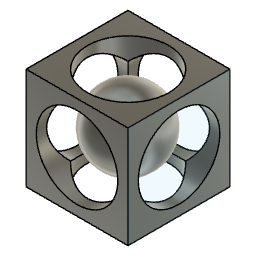
Sphere cube (Autodesk Fusion 360 design; units mm, degrees)
Autodesk Fusion 360 part; units mm, degrees
sketch "Sketch1" plane through (0, 0, 0) normal (0, 0, 1) x (1, 0, 0)
  line L0 (0, 25) -> (25, 25)
  line L1 (25, 25) -> (25, 0)
  line L2 (25, 0) -> (0, 0)
  line L3 (0, 0) -> (0, 25)
  constraint horizontal L0
  constraint perpendicular L0 L1
  constraint coincident L2.end L3.start
  constraint perpendicular L1 L2
  constraint perpendicular L0 L3
extrude "Extrude1" add sketch "Sketch1" along normal blind 25 makes body 1
sketch "Sketch2" plane through (0, 0, 0) normal (0, -1, 0) x (1, 0, 0)
  line L0 (0, 0) -> (25, 0)
  line L1 (25, 0) -> (25, 25)
  line L2 (25, 25) -> (0, 25)
  line L3 (0, 25) -> (0, 0)
  circle A0 centre (12.5, 12.5) radius 10
  dimension "d3" = 20
  measures "d3" diameter of A0
extrude "Extrude2" cut sketch "Sketch2" against normal blind 42 contours A0 bodies 1
sketch "Sketch3" plane through (25, 0, 0) normal (1, 0, 0) x (0, 1, 0)
  line L0 (0, 0) -> (25, 0)
  line L1 (25, 0) -> (25, 25)
  line L2 (25, 25) -> (0, 25)
  line L3 (0, 25) -> (0, 0)
sketch "Sketch4" plane through (25, 0, 0) normal (1, 0, 0) x (0, 1, 0)
  circle A0 centre (12.5309, 12.5169) radius 10
  dimension "d6" = 20
  measures "d6" diameter of A0
extrude "Extrude3" cut sketch "Sketch4" against normal blind 49 bodies 1
sketch "Sketch5" plane through (0, 0, 25) normal (0, 0, 1) x (-1, 0, 0)
  line L0 (0, 0) -> (-25, 0)
  line L1 (-25, 0) -> (-25, -25)
  line L2 (-25, -25) -> (0, -25)
  line L3 (0, -25) -> (0, 0)
  circle A0 centre (-12.5137, -12.5343) radius 10
  dimension "d9" = 20
  measures "d9" diameter of A0
extrude "Extrude4" cut sketch "Sketch5" against normal blind 40 contours A0 bodies 1
sketch "Sketch6" plane through (0, 0, 0) normal (0, 0, 1) x (1, 0, 0)
sphere "SpherePrimitive1" add diameter 18 placed x (1, 0, 0) y (0, 1, 0) z (0, 0, 1) at (-23, 7, 0) separate body makes body 2
move_body "Move1" bodies 2 to x (1, 0, 0) y (0, 1, 0) z (0, 0, 1) at (35.7487, 15.1625, 13)
move_body "MoveFace1" bodies 2 to x (1, 0, 0) y (0, 1, 0) z (0, 0, 1) at (0, -10, 0) on bodies 2
